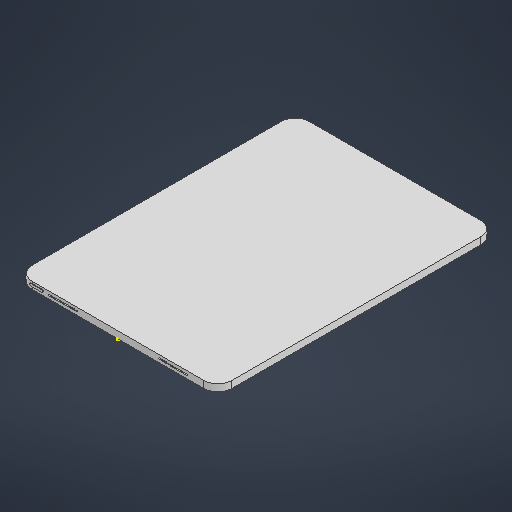
# Autodesk Inventor part: ipad
Saved by Autodesk Inventor 2026.2 (Build 302298000, 298)
## iProperties
Created: 2025-12-13
Part Number: ipad
Material: Generic
Document SubType Name: Modeling
Designer: 18705
Density: 1 g/cm^3
Appearance: Default
Author: 18705
Autodesk Inventor part; units mm, degrees
ref_plane "YZ Plane" through (0, 0, 0) normal (1, 0, 0) x (0, 1, 0)
ref_plane "XZ Plane" through (0, 0, 0) normal (0, 1, 0) x (-1, 0, 0)
ref_plane "XY Plane" through (0, 0, 0) normal (0, 0, 1) x (1, 0, 0)
sketch "Sketch2" plane through (0, 0, 0) normal (0, 1, 0) x (-1, 0, 0)
  line L0 (89, 123.5) -> (-89, 123.5)
  line L1 (-89, 123.5) -> (-89, -123.5)
  line L2 (-89, -123.5) -> (89, -123.5)
  line L3 (89, -123.5) -> (89, 123.5)
  line L4 (89, 123.5) -> (-89, -123.5) construction
  line L5 (-89, 123.5) -> (89, -123.5) construction
  point P0 (0, 0)
  dimension "d0" = 178
  dimension "d1" = 247
  constraints: 12 end point, 2 midpoint, 2 parallel, 1 horizontal, 1 perpendicular
  measures "d0" distance of L2.end L1.end
  measures "d1" distance of L1.end L0.end
extrude "Extrusion1" add sketch "Sketch2" along normal blind 6.22
fillet "Fillet1" radius 12.5 4 edges at (89, 3.11, 123.5) (-89, 3.11, 123.5) (-89, 3.11, -123.5) (89, 3.11, -123.5)
sketch "Sketch3" plane through (76.5, 0, 123.5) normal (0, 0, 1) x (1, 0, 0)
  point P0 (-76.5, 0)
sketch "Sketch4" plane through (76.5, 0, 123.5) normal (0, 0, 1) x (1, 0, 0)
  point P0 (-76.5, 0)
sketch "Sketch5" plane through (0, 0, 0) normal (0, -1, 0) x (1, 0, 0)
  line L0 (-83, 91.5) -> (-57, 91.5)
  line L1 (-57, 91.5) -> (-57, 117.5)
  line L2 (-57, 117.5) -> (-83, 117.5)
  line L3 (-83, 117.5) -> (-83, 91.5)
  line L4 (-83, 91.5) -> (-57, 117.5) construction
  line L5 (-57, 91.5) -> (-83, 117.5) construction
  line L6 (-89, 123.5) -> (76.5, 123.5) projected
  line L7 (-89, -123.5) -> (-89, 123.5) projected
  point P0 (0, 0)
  point P1 (-70, 104.5)
  point P2 (-76.3, 123.5)
  point P3 (-89, -110.8)
  point P4 (-89, 110.8)
  dimension "d8" = 26
  dimension "d9" = 26
  dimension "d10" = 6
  dimension "d11" = 6
  constraints: 12 end point, 2 midpoint, 2 parallel, 1 horizontal, 1 perpendicular
  measures "d8" distance of L2.end L1.end
  measures "d9" distance of L1.end L0.end
  measures "d10" distance between parallel lines of L2 L6
  measures "d11" distance between parallel lines of L7 L3
extrude "Extrusion2" add sketch "Sketch5" along normal blind 1.5
fillet "Fillet5" radius 4.7625 1 edges at (-83, -0.75, 91.5)
fillet "Fillet6" radius 4.7625 1 edges at (-57, -0.75, 91.5)
fillet "Fillet7" radius 4.7625 1 edges at (-57, -0.75, 117.5)
fillet "Fillet8" radius 4.7625 1 edges at (-83, -0.75, 117.5)
sketch "Sketch6" plane through (0, -1.5, 0) normal (0, -1, 0) x (1, 0, 0)
  circle A0 centre (-76, 110.4896) radius 5
  line L0 (-83, 112.7375) -> (-83, 96.2625) projected
  line L1 (-61.7625, 117.5) -> (-78.2375, 117.5) projected
  circle A1 centre (-76, 98.4896) radius 5
  point P0 (0, 0)
  dimension "d18" = 10
  dimension "d19" = 7
  dimension "d20" = 7.0104
  dimension "d23" = 12
  constraints: 2 centre point, 1 vertical, 2 other
  measures "d18" diameter of A0
  measures "d19" distance from line of L0 A0.centre
  measures "d20" distance from line of L1 A0.centre
  measures "d23" distance of A0.centre A1.centre
extrude "Extrusion3" add sketch "Sketch6" along normal blind 0.1
sketch "Sketch7" plane through (-76.5, 0, 123.5) normal (0, 0, 1) x (1, 0, 0)
  circle A0 centre (137.5, 3.11) radius 0.75
  line L0 (165.5, 0) -> (165.5, 6.22) projected
  line L1 (-12.5, 6.22) -> (-12.5, 0) projected
  line L2 (165.5, 3.11) -> (-12.5, 3.11) construction
  circle A1 centre (135.5, 3.11) radius 0.75
  circle A2 centre (133.5, 3.11) radius 0.75
  circle A3 centre (131.5, 3.11) radius 0.75
  circle A4 centre (129.5, 3.11) radius 0.75
  circle A5 centre (127.5, 3.11) radius 0.75
  circle A6 centre (125.5, 3.11) radius 0.75
  circle A7 centre (123.5, 3.11) radius 0.75
  circle A8 centre (121.5, 3.11) radius 0.75
  circle A9 centre (119.5, 3.11) radius 0.75
  circle A10 centre (117.5, 3.11) radius 0.75
  circle A11 centre (115.5, 3.11) radius 0.75
  circle A12 centre (113.5, 3.11) radius 0.75
  line L3 (153, 6.22) -> (153, 0) projected
  line L4 (0, 0) -> (0, 6.22) projected
  line L5 (0, 0) -> (153, 0) projected
  line L6 (0, 6.22) -> (153, 6.22) projected
  line L7 (76.5, 0) -> (76.5, 6.22) construction
  circle A13 centre (15.5, 3.11) radius 0.75
  circle A14 centre (17.5, 3.11) radius 0.75
  circle A15 centre (19.5, 3.11) radius 0.75
  circle A16 centre (21.5, 3.11) radius 0.75
  circle A17 centre (23.5, 3.11) radius 0.75
  circle A18 centre (25.5, 3.11) radius 0.75
  circle A19 centre (27.5, 3.11) radius 0.75
  circle A20 centre (29.5, 3.11) radius 0.75
  circle A21 centre (31.5, 3.11) radius 0.75
  circle A22 centre (33.5, 3.11) radius 0.75
  circle A23 centre (35.5, 3.11) radius 0.75
  circle A24 centre (37.5, 3.11) radius 0.75
  circle A25 centre (39.5, 3.11) radius 0.75
  dimension "d30" = 1.5
  dimension "d31" = 28
  dimension "d34" = 2
  constraints: 26 centre point, 13 symmetric about line, 4 end point, 3 midpoint, 1 horizontal, 1 point on line, 37 other
  measures "d30" diameter of A0
  measures "d31" distance from line of A0.centre L0
  measures "d34" distance of A0.centre A1.centre
extrude "Extrusion4" cut sketch "Sketch7" against normal blind 1 contours A0 | A1 | A2 | A3 | A4 | A5 | A6 | A7 | A8 | A9 | A10 | A11 | A12 | A13 | A14 | A15 | A16 | A17 | A18 | A19 | A20 | A21 | A22 | A23 | A24 | A25
sketch "Sketch8" plane through (76.5, 0, -123.5) normal (0, 0, -1) x (-1, 0, 0)
  circle A0 centre (137.5, 3.11) radius 0.75 projected
  circle A1 centre (135.5, 3.11) radius 0.75 projected
  circle A2 centre (133.5, 3.11) radius 0.75 projected
  circle A3 centre (131.5, 3.11) radius 0.75 projected
  circle A4 centre (129.5, 3.11) radius 0.75 projected
  circle A5 centre (127.5, 3.11) radius 0.75 projected
  circle A6 centre (125.5, 3.11) radius 0.75 projected
  circle A7 centre (123.5, 3.11) radius 0.75 projected
  circle A8 centre (121.5, 3.11) radius 0.75 projected
  circle A9 centre (119.5, 3.11) radius 0.75 projected
  circle A10 centre (117.5, 3.11) radius 0.75 projected
  circle A11 centre (115.5, 3.11) radius 0.75 projected
  circle A12 centre (113.5, 3.11) radius 0.75 projected
  circle A13 centre (39.5, 3.11) radius 0.75 projected
  circle A14 centre (37.5, 3.11) radius 0.75 projected
  circle A15 centre (35.5, 3.11) radius 0.75 projected
  circle A16 centre (33.5, 3.11) radius 0.75 projected
  circle A17 centre (31.5, 3.11) radius 0.75 projected
  circle A18 centre (29.5, 3.11) radius 0.75 projected
  circle A19 centre (27.5, 3.11) radius 0.75 projected
  circle A20 centre (25.5, 3.11) radius 0.75 projected
  circle A21 centre (23.5, 3.11) radius 0.75 projected
  circle A22 centre (21.5, 3.11) radius 0.75 projected
  circle A23 centre (19.5, 3.11) radius 0.75 projected
  circle A24 centre (17.5, 3.11) radius 0.75 projected
  circle A25 centre (15.5, 3.11) radius 0.75 projected
  line L0 (0, 6.22) -> (153, 6.22) projected
  line L1 (0, 0) -> (0, 6.22) projected
  line L2 (0, 0) -> (153, 0) projected
  line L3 (153, 6.22) -> (153, 0) projected
  line L4 (0, 6.22) -> (153, 6.22) projected
  point P0 (76.5, 0)
extrude "Extrusion5" cut sketch "Sketch8" against normal blind 1 contours A0 | A1 | A2 | A3 | A4 | A5 | A6 | A7 | A8 | A9 | A10 | A11 | A12 | A13 | A14 | A15 | A16 | A17 | A18 | A19 | A20 | A21 | A22 | A23 | A24 | A25
sketch "Sketch9" plane through (76.5, 0, -123.5) normal (0, 0, -1) x (-1, 0, 0)
  line L0 (0, 6.22) -> (153, 6.22) projected
  line L1 (0, 0) -> (153, 0) projected
  line L2 (76.5, 0) -> (76.5, 6.22) construction
  line L3 (72, 3.11) -> (81, 3.11)
  line L4 (73.25, 1.86) -> (79.75, 1.86)
  line L5 (79.75, 4.36) -> (73.25, 4.36)
  arc A0 (73.25, 4.36) -> (73.25, 1.86) centre (73.25, 3.11) ccw
  arc A1 (79.75, 1.86) -> (79.75, 4.36) centre (79.75, 3.11) ccw
  point P0 (76.5, 3.11)
  dimension "d43" = 9
  dimension "d44" = 2.5
  constraints: 10 end point, 6 point on circle, 4 tangent, 3 midpoint, 2 centre point, 2 point on line, 1 horizontal, 1 parallel
  measures "d43" distance of L3.start L3.end
  measures "d44" diameter of A1
extrude "Extrusion6" cut sketch "Sketch9" against normal blind 29.575
sketch "Sketch10" plane through (-76.5, 0, 123.5) normal (0, 0, 1) x (1, 0, 0)
  line L0 (-12.5, 6.22) -> (-12.5, 0) projected
  line L1 (165.5, 0) -> (165.5, 6.22) projected
  line L2 (-2, 3.4593) -> (10, 3.4593) construction
  line L3 (-1, 2.4593) -> (9, 2.4593)
  line L4 (9, 4.4593) -> (-1, 4.4593)
  arc A0 (-1, 4.4593) -> (-1, 2.4593) centre (-1, 3.4593) ccw
  arc A1 (9, 2.4593) -> (9, 4.4593) centre (9, 3.4593) ccw
  point P0 (76.5, 0)
  point P1 (4, 3.4593)
  dimension "d47" = 12
  dimension "d48" = 2
  dimension "d49" = 16.5
  constraints: 8 end point, 6 point on circle, 4 tangent, 2 centre point, 2 point on line, 1 horizontal, 1 midpoint, 1 parallel
  measures "d47" distance of L2.start L2.end
  measures "d48" diameter of A1
  measures "d49" distance from line of point (4, 3.459) L0
extrude "Extrusion7" add sketch "Sketch10" along normal blind 0.5
sketch "Sketch11" plane through (-89, 0, -111) normal (-1, 0, 0) x (0, 0, 1)
  line L0 (234.5, 0) -> (234.5, 2.4593) projected
  line L1 (234.5, 6.22) -> (222, 6.22) projected
  line L2 (222, 6.22) -> (222, 0) projected
  line L3 (222, 0) -> (234.5, 0) projected
  line L4 (234.5, 0) -> (234.5, 2.4593) projected
  line L5 (234.5, 2.4593) -> (234.5, 4.4593) projected
  line L6 (234.5, 4.4593) -> (234.5, 6.22) projected
  line L7 (234.5, 6.22) -> (234.5, 0) projected
  line L8 (234.5, 3.11) -> (-12.4159, 3.11) construction
  line L9 (214.5, 3.11) -> (205.5, 3.11) construction
  line L10 (213.25, 4.36) -> (206.75, 4.36)
  line L11 (206.75, 1.86) -> (213.25, 1.86)
  arc A0 (213.25, 1.86) -> (213.25, 4.36) centre (213.25, 3.11) ccw
  arc A1 (206.75, 4.36) -> (206.75, 1.86) centre (206.75, 3.11) ccw
  line L12 (202.25, 4.36) -> (195.75, 4.36)
  arc A2 (195.75, 4.36) -> (195.75, 1.86) centre (195.75, 3.11) ccw
  line L13 (195.75, 1.86) -> (202.25, 1.86)
  arc A3 (202.25, 1.86) -> (202.25, 4.36) centre (202.25, 3.11) ccw
  point P0 (111, 0)
  point P1 (210, 3.11)
  dimension "d52" = 9
  dimension "d53" = 2.5
  dimension "d54" = 24.5
  dimension "d57" = 11
  constraints: 14 end point, 10 point on circle, 4 centre point, 4 point on line, 4 tangent, 2 horizontal, 2 midpoint, 1 parallel, 10 other
  measures "d52" distance of L9.start L9.end
  measures "d53" diameter of A1
  measures "d54" distance from line of point (210, 3.11) L0
  measures "d57" distance of L10.start L12.start
extrude "Extrusion8" add sketch "Sketch11" along normal blind 0.5 contours A0 L11 A1 L10 | A3 L13 A2 L12
body "Solid1"
